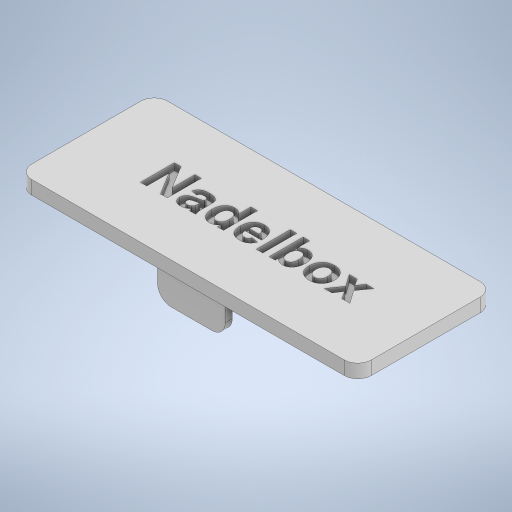
# Autodesk Inventor part: NadelboxDeckel
Saved by Autodesk Inventor 2023.1 (Build 271208000, 208)
## iProperties
Created: 2022-08-08
Part Number: NadelboxDeckel
Material: Generisch
Document SubType Name: Modeling
Designer: schwa
Density: 1 g/cm^3
Appearance: Vorgabe
Author: schwa
Autodesk Inventor part; units mm, degrees
note: some values were not read from the file. Chosen so that the rebuilt part matches the saved one: direction of "Prägen1".
ref_plane "YZ Plane" through (0, 0, 0) normal (1, 0, 0) x (0, 1, 0)
ref_plane "XZ Plane" through (0, 0, 0) normal (0, 1, 0) x (-1, 0, 0)
ref_plane "XY Plane" through (0, 0, 0) normal (0, 0, 1) x (1, 0, 0)
sketch "Skizze1" plane through (0, 0, 0) normal (0, 1, 0) x (-1, 0, 0)
  line L0 (25, 10) -> (-25, 10)
  line L1 (-25, 10) -> (-25, -10)
  line L2 (-25, -10) -> (25, -10)
  line L3 (25, -10) -> (25, 10)
  point P0 (0, 0)
  point P1 (0, -10)
  point P2 (-25, 0)
  dimension "d0" = 50
  dimension "d1" = 20
  dimension "d2" = 10
  dimension "d3" = 25
  constraints: 8 end point, 2 midpoint, 2 parallel, 1 horizontal, 1 perpendicular
  measures "d0" distance of L1.end L2.end
  measures "d1" distance of L1.end L0.end
  measures "d2" distance of point (0, -10) point (0, 0)
  measures "d3" distance of point (-25, 0) point (0, 0)
extrude "Extrusion1" add sketch "Skizze1" along normal blind 2
sketch "Skizze2" plane through (0, 0, 0) normal (0, -1, 0) x (1, 0, 0)
  line L0 (-5, 9.5) -> (5, 9.5)
  line L1 (5, 9.5) -> (5, 8.5)
  line L2 (5, 8.5) -> (-5, 8.5)
  line L3 (-5, 8.5) -> (-5, 9.5)
  line L4 (-5, -8.5) -> (5, -8.5)
  line L5 (5, -8.5) -> (5, -9.5)
  line L6 (5, -9.5) -> (-5, -9.5)
  line L7 (-5, -9.5) -> (-5, -8.5)
  line L8 (25, -10) -> (-25, -10) projected
  line L9 (-25, 10) -> (25, 10) projected
  point P0 (0, 0)
  point P1 (5, 9)
  dimension "d6" = 1
  dimension "d7" = 1
  dimension "d8" = 0.5
  dimension "d9" = 10
  dimension "d10" = 10
  dimension "d11" = 0.5
  dimension "d12" = 5
  constraints: 16 end point, 4 parallel, 2 horizontal, 2 perpendicular, 1 midpoint, 1 point on line
  measures "d6" distance of L1.end L0.end
  measures "d7" distance of L5.end L4.end
  measures "d8" distance between parallel lines of L8 L6
  measures "d9" distance of L4.end L4.start
  measures "d10" distance of L2.end L1.end
  measures "d11" distance between parallel lines of L9 L0
  measures "d12" horizontal distance of point (0, 0) point (5, 9)
extrude "Extrusion2" add sketch "Skizze2" along normal blind 4.5
fillet "Rundung1" radius 2 1 edges at (-5, -4.5, -9)
fillet "Rundung2" radius 2 3 edges at (5, -4.5, -9) (5, -4.5, 9) (-5, -4.5, 9)
fillet "Rundung3" radius 2 4 edges at (-25, 1, -10) (-25, 1, 10) (25, 1, 10) (25, 1, -10)
sketch "Skizze3" plane through (0, 2, 0) normal (0, 1, 0) x (1, 0, 0)
  line L0 (-18.4576, 7.1527) -> (19.5486, 7.1527) construction
  line L1 (19.5486, 7.1527) -> (19.5486, -6.9708) construction
  line L2 (19.5486, -6.9708) -> (-18.4576, -6.9708) construction
  line L3 (-18.4576, -6.9708) -> (-18.4576, 7.1527) construction
  line L4 (-14.6564, -2.3691) -> (-14.6564, 2.6309)
  line L5 (-14.6564, 2.6309) -> (-13.677, 2.6309)
  line L6 (-13.677, 2.6309) -> (-11.6229, -0.7227)
  line L7 (-11.6229, -0.7227) -> (-11.6229, 2.6309)
  line L8 (-11.6229, 2.6309) -> (-10.6892, 2.6309)
  line L9 (-10.6892, 2.6309) -> (-10.6892, -2.3691)
  line L10 (-10.6892, -2.3691) -> (-11.6991, -2.3691)
  line L11 (-11.6991, -2.3691) -> (-13.7227, 0.9122)
  line L12 (-13.7227, 0.9122) -> (-13.7227, -2.3691)
  line L13 (-13.7227, -2.3691) -> (-14.6564, -2.3691)
  line L14 (-8.9133, 0.15) -> (-9.7822, 0.3062)
  spline S0 degree 2 poles (-9.7822, 0.3062) (-9.6336, 0.8322) (-8.9171, 1.3352) (-8.2121, 1.3352) knots 0 0 0 1 2 2 2
  spline S1 degree 2 poles (-8.2121, 1.3352) (-7.568, 1.3352) (-6.9392, 1.0303) (-6.6839, 0.5654) (-6.6839, -0.0596) knots 0 0 0 1 2 3 3 3
  line L15 (-6.6839, -0.0596) -> (-6.6991, -1.18)
  spline S2 degree 2 poles (-6.6991, -1.18) (-6.6991, -1.6564) (-6.6077, -2.1099) (-6.4819, -2.3691) knots 0 0 0 1 2 2 2
  line L16 (-6.4819, -2.3691) -> (-7.4308, -2.3691)
  spline S3 degree 2 poles (-7.4308, -2.3691) (-7.4689, -2.2738) (-7.5223, -2.087) knots 0 0 0 1 1 1
  spline S4 degree 2 poles (-7.5223, -2.087) (-7.5452, -1.9994) (-7.5566, -1.9727) knots 0 0 0 1 1 1
  spline S5 degree 2 poles (-7.5566, -1.9727) (-7.8005, -2.209) (-8.3607, -2.4491) (-8.677, -2.4491) knots 0 0 0 1 2 2 2
  spline S6 degree 2 poles (-8.677, -2.4491) (-9.2372, -2.4491) (-9.8813, -1.8431) (-9.8813, -1.3782) knots 0 0 0 1 2 2 2
  spline S7 degree 2 poles (-9.8813, -1.3782) (-9.8813, -1.0695) (-9.5878, -0.5893) (-9.0581, -0.334) (-8.5589, -0.2387) knots 0 0 0 1 2 3 3 3
  spline S8 degree 2 poles (-8.5589, -0.2387) (-7.8881, -0.113) (-7.629, -0.0024) knots 0 0 0 1 1 1
  line L17 (-7.629, -0.0024) -> (-7.629, 0.0928)
  spline S9 degree 2 poles (-7.629, 0.0928) (-7.629, 0.3672) (-7.9034, 0.6035) (-8.2807, 0.6035) knots 0 0 0 1 2 2 2
  spline S10 degree 2 poles (-8.2807, 0.6035) (-8.536, 0.6035) (-8.8256, 0.4015) (-8.9133, 0.15) knots 0 0 0 1 2 2 2
  spline S11 degree 2 poles (-7.629, -0.6274) (-7.8119, -0.6884) (-8.6122, -0.8599) (-8.7342, -0.9399) knots 0 0 0 1 2 2 2
  spline S12 degree 2 poles (-8.7342, -0.9399) (-8.9209, -1.0733) (-8.9209, -1.2791) knots 0 0 0 1 1 1
  spline S13 degree 2 poles (-8.9209, -1.2791) (-8.9209, -1.4811) (-8.6199, -1.7745) (-8.3874, -1.7745) knots 0 0 0 1 2 2 2
  spline S14 degree 2 poles (-8.3874, -1.7745) (-8.1282, -1.7745) (-7.8958, -1.6031) knots 0 0 0 1 1 1
  spline S15 degree 2 poles (-7.8958, -1.6031) (-7.7205, -1.4735) (-7.6671, -1.2867) knots 0 0 0 1 1 1
  spline S16 degree 2 poles (-7.6671, -1.2867) (-7.629, -1.1648) (-7.629, -0.818) knots 0 0 0 1 1 1
  line L18 (-7.629, -0.818) -> (-7.629, -0.6274)
  line L19 (-2.4194, -2.3691) -> (-3.3112, -2.3691)
  line L20 (-3.3112, -2.3691) -> (-3.3112, -1.8355)
  spline S17 degree 2 poles (-3.3112, -1.8355) (-3.5322, -2.148) (-4.1381, -2.4491) (-4.443, -2.4491) knots 0 0 0 1 2 2 2
  spline S18 degree 2 poles (-4.443, -2.4491) (-5.068, -2.4491) (-5.9598, -1.443) (-5.9598, -0.5436) knots 0 0 0 1 2 2 2
  spline S19 degree 2 poles (-5.9598, -0.5436) (-5.9598, 0.3787) (-5.0947, 1.3352) (-4.4316, 1.3352) knots 0 0 0 1 2 2 2
  spline S20 degree 2 poles (-4.4316, 1.3352) (-3.8218, 1.3352) (-3.3798, 0.8322) knots 0 0 0 1 1 1
  line L21 (-3.3798, 0.8322) -> (-3.3798, 2.6309)
  line L22 (-3.3798, 2.6309) -> (-2.4194, 2.6309)
  line L23 (-2.4194, 2.6309) -> (-2.4194, -2.3691)
  spline S21 degree 2 poles (-4.9766, -0.4788) (-4.9766, -1.0581) (-4.8165, -1.3172) knots 0 0 0 1 1 1
  spline S22 degree 2 poles (-4.8165, -1.3172) (-4.584, -1.6907) (-4.1686, -1.6907) knots 0 0 0 1 1 1
  spline S23 degree 2 poles (-4.1686, -1.6907) (-3.8409, -1.6907) (-3.3759, -1.1267) (-3.3759, -0.5703) knots 0 0 0 1 2 2 2
  spline S24 degree 2 poles (-3.3759, -0.5703) (-3.3759, 0.0547) (-3.8256, 0.6035) (-4.1763, 0.6035) knots 0 0 0 1 2 2 2
  spline S25 degree 2 poles (-4.1763, 0.6035) (-4.5154, 0.6035) (-4.9766, 0.0623) (-4.9766, -0.4788) knots 0 0 0 1 2 2 2
  line L24 (0.6218, -1.2143) -> (1.5783, -1.3744)
  spline S26 degree 2 poles (1.5783, -1.3744) (1.3954, -1.9003) (0.5989, -2.4491) (0.0006, -2.4491) knots 0 0 0 1 2 2 2
  spline S27 degree 2 poles (0.0006, -2.4491) (-0.9445, -2.4491) (-1.3981, -1.8317) knots 0 0 0 1 1 1
  spline S28 degree 2 poles (-1.3981, -1.8317) (-1.7563, -1.3363) (-1.7563, -0.5855) knots 0 0 0 1 1 1
  spline S29 degree 2 poles (-1.7563, -0.5855) (-1.7563, 0.3177) (-0.815, 1.3352) (-0.0947, 1.3352) knots 0 0 0 1 2 2 2
  spline S30 degree 2 poles (-0.0947, 1.3352) (0.7132, 1.3352) (1.6469, 0.2681) (1.6279, -0.8332) knots 0 0 0 1 2 2 2
  line L25 (1.6279, -0.8332) -> (-0.7731, -0.8332)
  spline S31 degree 2 poles (-0.7731, -0.8332) (-0.7616, -1.2601) (-0.3195, -1.7326) (0.012, -1.7326) knots 0 0 0 1 2 2 2
  spline S32 degree 2 poles (0.012, -1.7326) (0.2369, -1.7326) (0.5417, -1.4887) (0.6218, -1.2143) knots 0 0 0 1 2 2 2
  spline S33 degree 2 poles (0.6751, -0.2463) (0.6637, 0.169) (0.2559, 0.6035) (-0.0375, 0.6035) knots 0 0 0 1 2 2 2
  spline S34 degree 2 poles (-0.0375, 0.6035) (-0.35, 0.6035) (-0.5558, 0.3748) knots 0 0 0 1 1 1
  spline S35 degree 2 poles (-0.5558, 0.3748) (-0.7578, 0.1462) (-0.7578, -0.2463) knots 0 0 0 1 1 1
  line L26 (-0.7578, -0.2463) -> (0.6751, -0.2463)
  line L27 (2.4091, -2.3691) -> (2.4091, 2.6309)
  line L28 (2.4091, 2.6309) -> (3.3695, 2.6309)
  line L29 (3.3695, 2.6309) -> (3.3695, -2.3691)
  line L30 (3.3695, -2.3691) -> (2.4091, -2.3691)
  line L31 (4.307, -2.3691) -> (4.307, 2.6309)
  line L32 (4.307, 2.6309) -> (5.2673, 2.6309)
  line L33 (5.2673, 2.6309) -> (5.2673, 0.8322)
  spline S36 degree 2 poles (5.2673, 0.8322) (5.7094, 1.3352) (6.3154, 1.3352) knots 0 0 0 1 1 1
  spline S37 degree 2 poles (6.3154, 1.3352) (6.9785, 1.3352) (7.8436, 0.3787) (7.8436, -0.5207) knots 0 0 0 1 2 2 2
  spline S38 degree 2 poles (7.8436, -0.5207) (7.8436, -1.4468) (6.9594, -2.4491) (6.3306, -2.4491) knots 0 0 0 1 2 2 2
  spline S39 degree 2 poles (6.3306, -2.4491) (6.0219, -2.4491) (5.416, -2.1404) (5.1987, -1.8355) knots 0 0 0 1 2 2 2
  line L34 (5.1987, -1.8355) -> (5.1987, -2.3691)
  line L35 (5.1987, -2.3691) -> (4.307, -2.3691)
  spline S40 degree 2 poles (5.2597, -0.4788) (5.2597, -1.039) (5.435, -1.3096) knots 0 0 0 1 1 1
  spline S41 degree 2 poles (5.435, -1.3096) (5.6866, -1.6907) (6.0981, -1.6907) knots 0 0 0 1 1 1
  spline S42 degree 2 poles (6.0981, -1.6907) (6.4144, -1.6907) (6.8603, -1.1495) (6.8603, -0.5665) knots 0 0 0 1 2 2 2
  spline S43 degree 2 poles (6.8603, -0.5665) (6.8603, 0.0547) (6.4106, 0.6035) (6.06, 0.6035) knots 0 0 0 1 2 2 2
  spline S44 degree 2 poles (6.06, 0.6035) (5.717, 0.6035) (5.2597, 0.07) (5.2597, -0.4788) knots 0 0 0 1 2 2 2
  spline S45 degree 2 poles (8.3923, -0.5055) (8.3923, -0.0291) (8.8649, 0.8665) (9.7262, 1.3352) (10.2597, 1.3352) knots 0 0 0 1 2 3 3 3
  spline S46 degree 2 poles (10.2597, 1.3352) (11.0829, 1.3352) (12.1347, 0.2681) (12.1347, -0.5474) knots 0 0 0 1 2 2 2
  spline S47 degree 2 poles (12.1347, -0.5474) (12.1347, -1.3668) (11.0715, -2.4491) (10.2673, -2.4491) knots 0 0 0 1 2 2 2
  spline S48 degree 2 poles (10.2673, -2.4491) (9.7681, -2.4491) (8.8649, -1.9994) (8.3923, -1.1305) (8.3923, -0.5055) knots 0 0 0 1 2 3 3 3
  spline S49 degree 2 poles (9.3756, -0.555) (9.3756, -1.0962) (9.8862, -1.6678) (10.2635, -1.6678) knots 0 0 0 1 2 2 2
  spline S50 degree 2 poles (10.2635, -1.6678) (10.6408, -1.6678) (11.1477, -1.0962) (11.1477, -0.5512) knots 0 0 0 1 2 2 2
  spline S51 degree 2 poles (11.1477, -0.5512) (11.1477, -0.0177) (10.6408, 0.554) (10.2635, 0.554) knots 0 0 0 1 2 2 2
  spline S52 degree 2 poles (10.2635, 0.554) (9.8862, 0.554) (9.3756, -0.0177) (9.3756, -0.555) knots 0 0 0 1 2 2 2
  line L36 (12.4244, -2.3691) -> (13.7277, -0.5017)
  line L37 (13.7277, -0.5017) -> (12.4777, 1.2552)
  line L38 (12.4777, 1.2552) -> (13.6477, 1.2552)
  line L39 (13.6477, 1.2552) -> (14.2879, 0.2605)
  line L40 (14.2879, 0.2605) -> (14.9625, 1.2552)
  line L41 (14.9625, 1.2552) -> (16.0867, 1.2552)
  line L42 (16.0867, 1.2552) -> (14.8596, -0.4598)
  line L43 (14.8596, -0.4598) -> (16.201, -2.3691)
  line L44 (16.201, -2.3691) -> (15.0234, -2.3691)
  line L45 (15.0234, -2.3691) -> (14.2879, -1.2448)
  line L46 (14.2879, -1.2448) -> (13.5448, -2.3691)
  line L47 (13.5448, -2.3691) -> (12.4244, -2.3691)
  point P0 (0, 0)
  constraints: 2 other
emboss "Prägen1" sketch "Skizze3" operation cut depth 1 direction (0, -1, 0)
